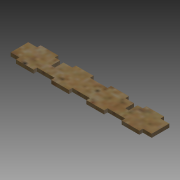
# Autodesk Inventor part: LongMiddleStructure
Saved by Autodesk Inventor 2012 (Build 160160000, 160)
## iProperties
Created: 2014-07-01
Part Number: LongMiddleStructure
Material: Default
Document SubType Name: Modeling
Designer: Laurent
Density: 1 g/cm^3
Author: Laurent
Autodesk Inventor part; units mm, degrees
ref_plane "YZ Plane" through (0, 0, 0) normal (1, 0, 0) x (0, 1, 0)
ref_plane "XZ Plane" through (0, 0, 0) normal (0, 1, 0) x (-1, 0, 0)
ref_plane "XY Plane" through (0, 0, 0) normal (0, 0, 1) x (1, 0, 0)
sketch "Sketch1" plane through (0, 0, 0) normal (0, 0, 1) x (1, 0, 0)
  line L0 (-80, 14) -> (80, 14)
  line L1 (80, 14) -> (80, -14)
  line L2 (80, -14) -> (-80, -14)
  line L3 (-80, -14) -> (-80, 14)
  point P0 (0, 0)
  dimension "d0" = 160
  dimension "d1" = 28
  dimension "d2" = 14
  dimension "d3" = 80
  constraints: 8 end point, 2 parallel, 1 horizontal, 1 perpendicular
  measures "d0" distance of L1.end L2.end
  measures "d1" distance of L0.end L1.end
  measures "d2" distance from line of L0 point (0, 0)
  measures "d3" distance from line of L1 point (0, 0)
extrude "Base" add sketch "Sketch1" along normal blind 4
sketch "Sketch2" plane through (0, 0, 4) normal (0, 0, 1) x (1, 0, 0)
  line L0 (-80, 14) -> (80, 14) projected
  line L1 (80, -14) -> (-80, -14) projected
  line L2 (-50, 14) -> (-30, 14)
  line L3 (-30, 14) -> (-30, 10)
  line L4 (-30, 10) -> (-50, 10)
  line L5 (-50, 10) -> (-50, 14)
  line L6 (-10, 14) -> (10, 14)
  line L7 (10, 14) -> (10, 10)
  line L8 (10, 10) -> (-10, 10)
  line L9 (-10, 10) -> (-10, 14)
  line L10 (30, 14) -> (50, 14)
  line L11 (50, 14) -> (50, 10)
  line L12 (50, 10) -> (30, 10)
  line L13 (30, 10) -> (30, 14)
  line L14 (-50, -10) -> (-30, -10)
  line L15 (-30, -10) -> (-30, -14)
  line L16 (-30, -14) -> (-50, -14)
  line L17 (-50, -14) -> (-50, -10)
  line L18 (-10, -10) -> (10, -10)
  line L19 (10, -10) -> (10, -14)
  line L20 (10, -14) -> (-10, -14)
  line L21 (-10, -14) -> (-10, -10)
  line L22 (30, -10) -> (50, -10)
  line L23 (50, -10) -> (50, -14)
  line L24 (50, -14) -> (30, -14)
  line L25 (30, -14) -> (30, -10)
  line L26 (80, 14) -> (80, -14) projected
  line L27 (-80, -14) -> (-80, 14) projected
  line L28 (-80, -10) -> (-70, -10)
  line L29 (-70, -10) -> (-70, -14)
  line L30 (-70, -14) -> (-80, -14)
  line L31 (-80, -14) -> (-80, -10)
  line L32 (-80, 14) -> (-70, 14)
  line L33 (-70, 14) -> (-70, 10)
  line L34 (-70, 10) -> (-80, 10)
  line L35 (-80, 10) -> (-80, 14)
  line L36 (70, 14) -> (80, 14)
  line L37 (80, 14) -> (80, 10)
  line L38 (80, 10) -> (70, 10)
  line L39 (70, 10) -> (70, 14)
  line L40 (70, -10) -> (80, -10)
  line L41 (80, -10) -> (80, -14)
  line L42 (80, -14) -> (70, -14)
  line L43 (70, -14) -> (70, -10)
  point P0 (0, 0)
  dimension "d6" = 20
  dimension "d7" = 4
  dimension "d10" = 40
  dimension "d19" = 20
  dimension "d20" = 4
  dimension "d21" = 40
  dimension "d25" = 0
  dimension "d40" = 4
  dimension "d42" = 10
  dimension "d43" = 10
  dimension "d44" = 10
  dimension "d45" = 4
  dimension "d54" = 10
  dimension "d55" = 4
  dimension "d64" = 10
  dimension "d65" = 4
  dimension "d74" = 10
  dimension "d75" = 4
  dimension "d76" = 0
  dimension "d77" = 0
  dimension "d78" = 0
  dimension "d79" = 0
  dimension "d80" = 0
  dimension "d81" = 0
  dimension "d82" = 0
  dimension "d83" = 0
  constraints: 80 end point, 12 parallel, 8 horizontal, 6 perpendicular, 2 collinear, 30 other
  measures "d6" distance of L3.end L4.end
  measures "d7" distance of L2.end L3.end
  measures "d10" distance of L2.start L6.start
  measures "d19" distance of L15.end L16.end
  measures "d20" distance of L15.start L15.end
  measures "d21" distance of L14.start L18.start
  measures "d25" distance between parallel lines of L1 L16
  measures "d40" distance between parallel lines of L0 L8
  measures "d42" distance from line of point (0, 0) L21
  measures "d43" distance from line of point (0, 0) L9
  measures "d44" distance of L29.end L30.end
  measures "d45" distance of L28.end L29.end
  measures "d54" distance of L33.end L34.end
  measures "d55" distance of L32.end L33.end
  measures "d64" distance of L37.end L38.end
  measures "d65" distance of L36.end L37.end
  measures "d74" distance of L41.end L42.end
  measures "d75" distance of L40.end L41.end
  measures "d76" distance between parallel lines of L0 L32
  measures "d77" distance between parallel lines of L27 L35
  measures "d78" distance between parallel lines of L1 L30
  measures "d79" distance between parallel lines of L27 L31
  measures "d80" distance between parallel lines of L26 L41
  measures "d81" distance between parallel lines of L1 L42
  measures "d82" distance between parallel lines of L0 L36
  measures "d83" distance between parallel lines of L26 L37
extrude "Platformsleeves" cut sketch "Sketch2" against normal blind 4 contours L0 L33 L34 L27 | L0 L3 L4 L5 | L28 L29 L1 L27 | L0 L7 L8 L9 | L17 L14 L15 L1 | L0 L11 L12 L13 | L21 L18 L19 L1 | L0 L26 L38 L39 | L25 L22 L23 L1 | L26 L1 L43 L40
sketch "Sketch4" plane through (0, 0, 4) normal (0, 0, 1) x (1, 0, 0)
  line L0 (30, 10) -> (30, 14) projected
  line L1 (-30, 14) -> (-30, 10) projected
  line L2 (-30, 10) -> (-50, 10) projected
  line L3 (50, 10) -> (30, 10) projected
  line L4 (-44, 10) -> (-40, 10)
  line L5 (-40, 10) -> (-40, 0)
  line L6 (-40, 0) -> (-44, 0)
  line L7 (-44, 0) -> (-44, 10)
  line L8 (40, 10) -> (44, 10)
  line L9 (44, 10) -> (44, 0)
  line L10 (44, 0) -> (40, 0)
  line L11 (40, 0) -> (40, 10)
  point P0 (0, 0)
  dimension "d86" = 4
  dimension "d87" = 10
  dimension "d88" = 10
  dimension "d89" = 0
  dimension "d90" = 4
  dimension "d91" = 10
  dimension "d92" = 10
  dimension "d93" = 0
  constraints: 16 end point, 4 parallel, 2 horizontal, 2 perpendicular
  measures "d86" distance of L5.end L6.end
  measures "d87" distance of L4.end L5.end
  measures "d88" distance between parallel lines of L1 L5
  measures "d89" distance between parallel lines of L2 L4
  measures "d90" distance of L9.end L10.end
  measures "d91" distance of L8.end L9.end
  measures "d92" distance between parallel lines of L0 L11
  measures "d93" distance between parallel lines of L3 L8
extrude "Sleeves" cut sketch "Sketch4" against normal blind 4
body "Solid1"
